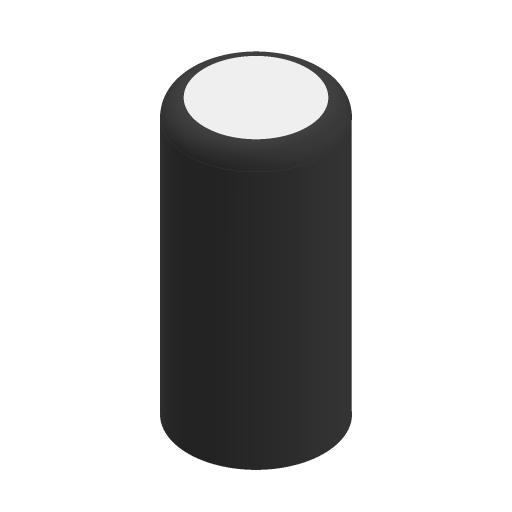
# Autodesk Inventor part: Capacitor
Saved by Autodesk Inventor 2024 (Build 280153000, 153)
## iProperties
Created: 2024-09-24
Part Number: Capacitor
Material: Generic
Document SubType Name: Modeling
Designer: Laith Al-Sadi
Density: 1 g/cm^3
Appearance: Default
Author: Laith Al-Sadi
Autodesk Inventor part; units mm, degrees
ref_plane "YZ Plane" through (0, 0, 0) normal (1, 0, 0) x (0, 1, 0)
ref_plane "XZ Plane" through (0, 0, 0) normal (0, 1, 0) x (-1, 0, 0)
ref_plane "XY Plane" through (0, 0, 0) normal (0, 0, 1) x (1, 0, 0)
sketch "Sketch1" plane through (0, 0, 0) normal (0, 1, 0) x (-1, 0, 0)
  circle A0 centre (0, 0) radius 2.05
  dimension "d0" = 4.1
  constraints: 1 centre point, 1 coincident
  measures "d0" diameter of A0
extrude "Extrusion1" add sketch "Sketch1" along normal blind 8.3
fillet "Fillet1" radius 0.5 1 edges at (2.05, 8.3, 0)
body "Solid1"
